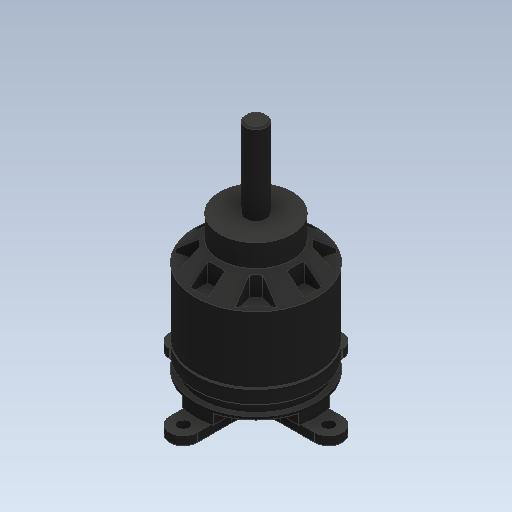
# Autodesk Inventor part: CobraCP2814-1050kv
Saved by Autodesk Inventor 2020 (Build 240168000, 168)
## iProperties
Part Number: CobraCP2814-1050kv
Material: GEDA Polyamid schwarz
Document SubType Name: Modeling
Designer: Admin
Mass: 32.8835 g
Surface Area: 99.7314 cm^2
Volume: 28.8452 cm^3
Density: 1.14 g/cm^3
Appearance: GEDA Plastik schwarz A
Gewicht: 0,033 kg
G_L: 0
G_H: 0
G_B: 0
InventorVersion: 2019.4
VAULT_Status: in Bearbeitung
Revision: -
Max. Breite: 0
Max. Höhe: 0
Max. Länge: 0
Max. Abmessungen: 0 x 0 x 0
Author: Admin
Autodesk Inventor part; units mm, degrees
note: some values were not read from the file. Left out: dimensions or parameters whose unit could not be read.
ref_plane "YZ Plane" through (0, 0, 0) normal (1, 0, 0) x (0, 1, 0)
ref_plane "XZ Plane" through (0, 0, 0) normal (0, 1, 0) x (-1, 0, 0)
ref_plane "XY Plane" through (0, 0, 0) normal (0, 0, 1) x (1, 0, 0)
sketch "Skizze1" plane through (0, 0, 0) normal (0, 0, 1) x (1, 0, 0)
  circle A0 centre (0, 0) radius 17.5
  dimension "d0" = 35
  constraints: 1 centre point, 1 coincident
  measures "d0" diameter of A0
extrude "Extrusion1" add sketch "Skizze1" along normal blind 36
sketch "Skizze3" plane through (0, 0, 36) normal (0, 0, 1) x (1, 0, 0)
  circle A0 centre (0, 0) radius 10.5
  dimension "d11" = 21
  constraints: 1 centre point, 1 coincident
  measures "d11" diameter of A0
chamfer "Fase2" distance 7 angle 40 1 edges at (-17.5, 0, 36) measured on face at (4.865, -5.1831, 36)
extrude "Extrusion2" add sketch "Skizze3" along normal blind 6.5
sketch "Skizze4" plane through (0, 0, 42.5) normal (0, 0, 1) x (1, 0, 0)
  circle A0 centre (0, 0) radius 3
  dimension "d17" = 6
  constraints: 1 centre point, 1 coincident
  measures "d17" diameter of A0
extrude "Extrusion3" add sketch "Skizze4" along normal blind 23.5
chamfer "Fase3" distance 0.5 angle 45 1 edges at (-3, 0, 66)
sketch "Skizze2" plane through (0, 0, 0) normal (1, 0, 0) x (0, 1, 0)
  line L0 (17.5, 11.1263) -> (16.5, 11.1263)
  line L1 (16.5, 11.1263) -> (16.5, 10.6263)
  line L2 (16.5, 10.6263) -> (17.5, 10.6263)
  line L3 (17.5, 10.6263) -> (17.5, 11.1263)
  line L4 (-17.5, 0) -> (17.5, 0) projected
  line L5 (17.5, 30.1263) -> (-17.5, 30.1263) projected
  point P0 (0, 0)
  point P1 (-17.5, 32)
  dimension "d6" = 1
  dimension "d7" = 0.5
  dimension "d23" = 19
  constraints: 8 end point, 2 parallel, 1 horizontal, 1 perpendicular, 1 point on line
  measures "d6" distance of L2.end L1.end
  measures "d7" distance of L1.end L0.end
  measures "d23" distance from line of L5 L0.start
sketch3d "3D-Skizze2"
  arc A0 (17.5, 0, 0) -> (0, -17.5, 0) centre (0, 0, 0) ccw
  arc A1 (0, -17.5, 0) -> (-17.5, 0, 0) centre (0, 0, 0) ccw
  arc A2 (-17.5, 0, 0) -> (0, 17.5, 0) centre (0, 0, 0) ccw
  arc A3 (0, 17.5, 0) -> (17.5, 0, 0) centre (0, 0, 0) ccw
sweep "Sweeping2" cut profiles "Skizze2" path "3D-Skizze2"
sketch "Skizze5" plane through (0, 0, 0) normal (0, 0, -1) x (-1, 0, 0)
  circle A0 centre (0, 0) radius 12.5 construction
  circle A1 centre (0, 12.5) radius 1.5
  circle A2 centre (12.5, 0) radius 1.5
  circle A3 centre (0, -12.5) radius 1.5
  circle A4 centre (-12.5, 0) radius 1.5
  dimension "d26" = 25
  dimension "d27" = 3
  constraints: 5 centre point, 4 point on circle, 3 equal radius, 2 horizontal alignment, 2 vertical alignment, 1 coincident
  measures "d26" diameter of A0
  measures "d27" diameter of A1
extrude "Extrusion4" cut sketch "Skizze5" against normal blind 5
sketch "Skizze6" plane through (0, 0, 0) normal (0, 0, -1) x (-1, 0, 0)
  line L0 (-4.5, -17.5) -> (4.5, -17.5) construction
  line L1 (4.5, -17.5) -> (4.5, 17.5) construction
  line L2 (4.5, 17.5) -> (-4.5, 17.5) construction
  line L3 (-4.5, 17.5) -> (-4.5, -17.5) construction
  line L4 (-4.5, -17.5) -> (4.5, 17.5) construction
  line L5 (4.5, -17.5) -> (-4.5, 17.5) construction
  line L6 (-17.5, -4.5) -> (17.5, -4.5) construction
  line L7 (17.5, -4.5) -> (17.5, 4.5) construction
  line L8 (17.5, 4.5) -> (-17.5, 4.5) construction
  line L9 (-17.5, 4.5) -> (-17.5, -4.5) construction
  line L10 (-17.5, -4.5) -> (17.5, 4.5) construction
  line L11 (17.5, -4.5) -> (-17.5, 4.5) construction
  circle A0 centre (0, 0) radius 17.5 projected
  circle A1 centre (0, 12.5) radius 1.5 construction
  circle A2 centre (12.5, 0) radius 1.5 construction
  circle A3 centre (0, -12.5) radius 1.5 construction
  circle A4 centre (-12.5, 0) radius 1.5 construction
  line L12 (0, -12.5) -> (12.5, 0) construction
  line L13 (12.5, 0) -> (0, 12.5) construction
  line L14 (0, 12.5) -> (-12.5, 0) construction
  line L15 (-12.5, 0) -> (0, -12.5) construction
  line L16 (0, -12.5) -> (0, 12.5) construction
  line L17 (12.5, 0) -> (-12.5, 0) construction
  circle A5 centre (0, 0) radius 17.5
  line L18 (-4.5, 16.9115) -> (-4.5, 8)
  line L19 (-4.5, 8) -> (-8, 4.5)
  line L20 (-16.9115, 4.5) -> (-8, 4.5)
  line L21 (4.5, 16.9115) -> (4.5, 8)
  line L22 (8, 4.5) -> (4.5, 8)
  line L23 (8, 4.5) -> (16.9115, 4.5)
  line L24 (-16.9115, -4.5) -> (-8, -4.5)
  line L25 (-8, -4.5) -> (-4.5, -8)
  line L26 (-4.5, -8) -> (-4.5, -16.9115)
  line L27 (4.5, -16.9115) -> (4.5, -8)
  line L28 (8, -4.5) -> (4.5, -8)
  line L29 (8, -4.5) -> (16.9115, -4.5)
  dimension "d31" = 9
  dimension "d32" = 9
  constraints: 60 end point, 24 point on line, 6 midpoint, 6 parallel, 4 perpendicular, 3 coincident, 2 collinear, 2 horizontal, 2 tangent, 11 other
  measures "d31" distance of L2.end L1.end
  measures "d32" distance of L7.end L6.end
extrude "Extrusion5" cut sketch "Skizze6" against normal blind 3 contours L23 L22 L21 A0 | A0 L27 L28 L29 | L18 L19 L20 A0 | A0 L24 L25 L26
fillet "Rundung1" radius 3 8 edges at (-8, 4.5, 1.5) (-4.5, 8, 1.5) (-8, -4.5, 1.5) (-4.5, -8, 1.5) (4.5, -8, 1.5) (8, -4.5, 1.5) (8, 4.5, 1.5) (4.5, 8, 1.5)
sketch "Skizze7" plane through (0, 0, 0) normal (1, 0, 0) x (0, 1, 0)
  line L0 (0, 1.5) -> (0, 10.6263)
  line L1 (0, 10.6263) -> (14.5, 10.6263)
  line L2 (9.2426, 3) -> (16.9115, 3) projected
  line L3 (14.5, 10.6263) -> (14.5, 1.5)
  line L4 (14.5, 1.5) -> (0, 1.5)
  line L5 (16.9115, 0) -> (9.2426, 0) projected
  line L6 (7.1213, 0) -> (9.2426, 0) projected
  line L7 (7.1213, 0) -> (5.3787, 0) projected
  line L8 (4.5, 0) -> (5.3787, 0) projected
  line L9 (-5.3787, 0) -> (-4.5, 0) projected
  line L10 (-5.3787, 0) -> (-7.1213, 0) projected
  line L11 (-9.2426, 0) -> (-7.1213, 0) projected
  line L12 (-9.2426, 0) -> (-16.9115, 0) projected
  line L13 (-16.9115, 0) -> (-9.2426, 0) projected
  line L14 (-7.1213, 0) -> (-9.2426, 0) projected
  line L15 (-7.1213, 0) -> (-5.3787, 0) projected
  line L16 (-4.5, 0) -> (-5.3787, 0) projected
  line L17 (5.3787, 0) -> (4.5, 0) projected
  line L18 (5.3787, 0) -> (7.1213, 0) projected
  line L19 (9.2426, 0) -> (7.1213, 0) projected
  line L20 (9.2426, 0) -> (16.9115, 0) projected
  line L21 (1.5, 0) -> (-1.5, 0) projected
  line L22 (1.5, 0) -> (-1.5, 0) projected
  line L23 (14, 0) -> (11, 0) projected
  line L24 (-11, 0) -> (-14, 0) projected
  line L25 (-17.5, 10.6263) -> (17.5, 10.6263) projected
  line L26 (-16.9115, 0) -> (-16.9115, 0) projected
  line L27 (-4.5, 0) -> (4.5, 0) projected
  line L28 (16.9115, 0) -> (16.9115, 0) projected
  line L29 (4.5, 0) -> (-4.5, 0) projected
  line L30 (17.5, 0) -> (17.5, 10.6263) projected
  line L31 (16, 3.8132) -> (17.5, 3.8132)
  line L32 (17.5, 3.8132) -> (17.5, 6.8132)
  line L33 (17.5, 6.8132) -> (16, 6.8132)
  line L34 (16, 6.8132) -> (16, 3.8132)
  line L35 (16, 3.8132) -> (17.5, 6.8132) construction
  line L36 (17.5, 3.8132) -> (16, 6.8132) construction
  point P0 (0, 0)
  point P1 (16.691, 9)
  point P2 (16.75, 5.3132)
  point P3 (16.75, 5.3132)
  point P4 (17.5, 5.3132)
  dimension "d41" = 1.5
  dimension "d75" = 3
  dimension "d76" = 1.5
  dimension "d77" = 3
  constraints: 20 end point, 4 midpoint, 4 parallel, 2 collinear, 2 horizontal, 1 horizontal alignment, 1 perpendicular, 1 point on line, 1 vertical, 1 other
  measures "d41" distance between parallel lines of L19 L4
  measures "d75" distance between parallel lines of L3 L30
  measures "d76" distance of L33.end L32.end
  measures "d77" distance of L33.end L31.start
revolve "Umdrehung1" cut sketch "Skizze7" angle 360 about axis through (0, 0, 1.5) along (0, 0, 1)
sketch "Skizze8" plane through (0, 0, 42.5) normal (0, 0, 1) x (1, 0, 0)
  circle A0 centre (0, 0) radius 17.5 projected
  circle A1 centre (0, 0) radius 10.5 projected
  line L0 (-2.5, 11.5) -> (2.5, 11.5)
  line L1 (2.5, 11.5) -> (2.5, 16.5)
  line L2 (2.5, 16.5) -> (-2.5, 16.5)
  line L3 (-2.5, 16.5) -> (-2.5, 11.5)
  line L4 (-2.5, 11.5) -> (2.5, 16.5) construction
  line L5 (2.5, 11.5) -> (-2.5, 16.5) construction
  line L6 (8.626, 14.7085) -> (14.7085, 8.626)
  line L7 (14.7085, 8.626) -> (9.1317, 7.1317)
  line L8 (9.1317, 7.1317) -> (7.1317, 9.1317)
  line L9 (7.1317, 9.1317) -> (8.626, 14.7085)
  line L10 (0, 0) -> (8.1317, 8.1317) construction
  line L11 (0, 0) -> (0, 14) construction
  dimension "d11" = 21
  dimension "d43" = 14
  dimension "d44" = 5
  dimension "d45" = 5
  dimension "d46" = 30
  dimension "d47" = 45
  dimension "d48" = 11.5
  dimension "d49" = 11.5
  dimension "d50" = 16.5
  dimension "d51" = 16.5
  dimension "d78" = 2
  constraints: 24 end point, 3 midpoint, 2 parallel, 2 perpendicular, 1 coincident, 1 horizontal, 1 vertical, 1 other
  measures "d43" distance of point (0, 0) L11.end
  measures "d44" distance of L0.end L1.end
  measures "d45" distance of L0.start L0.end
  measures "d46" angle of L9 L10
  measures "d47" angle of L11 L10
  measures "d48" distance from line of point (0, 0) L0
  measures "d49" distance from line of L8 point (0, 0)
  measures "d50" distance from line of L2 point (0, 0)
  measures "d51" distance from line of point (0, 0) L6
  measures "d78" horizontal distance of L7.end L8.end
extrude "Extrusion6" cut sketch "Skizze8" against normal blind 13 contours L3 L2 L1 L0 | L6 L7 L8 L9
pattern_circular "Runde Anordnung1" count 4 over 360 about axis through (0, 0, -10) along (0, 0, 1) of "Extrusion6"
sketch "Skizze9" plane through (0, 0, 0) normal (0, 0, -1) x (-1, 0, 0)
  line L0 (-4, 25) -> (4, 25)
  line L1 (4, 25) -> (4, -25)
  line L2 (4, -25) -> (-4, -25)
  line L3 (-4, -25) -> (-4, 25)
  line L4 (-4, 25) -> (4, -25) construction
  line L5 (4, 25) -> (-4, -25) construction
  line L6 (-25, 4) -> (25, 4)
  line L7 (25, 4) -> (25, -4)
  line L8 (25, -4) -> (-25, -4)
  line L9 (-25, -4) -> (-25, 4)
  line L10 (-25, 4) -> (25, -4) construction
  line L11 (25, 4) -> (-25, -4) construction
  circle A0 centre (21, 0) radius 1.65
  circle A1 centre (0, 21) radius 1.65
  circle A2 centre (-21, 0) radius 1.65
  circle A3 centre (0, -21) radius 1.65
  line L12 (21, 0) -> (0, -21) construction
  line L13 (0, 21) -> (-21, 0) construction
  circle A4 centre (0, 12.5) radius 1.5 projected
  circle A5 centre (12.5, 0) radius 1.5 projected
  circle A6 centre (0, -12.5) radius 1.5 projected
  circle A7 centre (-12.5, 0) radius 1.5 projected
  point P0 (0, 0)
  dimension "d57" = 8
  dimension "d58" = 50
  dimension "d59" = 50
  dimension "d60" = 8
  dimension "d61" = 3.3
  dimension "d64" = 360
  dimension "d67" = 42
  constraints: 28 end point, 4 centre point, 4 midpoint, 4 parallel, 2 horizontal, 2 perpendicular, 9 other
  measures "d57" distance of L1.end L2.end
  measures "d58" distance of L0.end L1.end
  measures "d59" distance of L7.end L8.end
  measures "d60" distance of L6.end L7.end
  measures "d61" diameter of A0
  measures "d67" distance of L13.end L12.start
extrude "Extrusion7" add sketch "Skizze9" along normal blind 2.5
fillet "Rundung3" radius 7 4 edges at (-4, -4, -1.25) (-4, 4, -1.25) (4, 4, -1.25) (4, -4, -1.25)
fillet "Rundung4" radius 4 8 edges at (-25, -4, -1.25) (-25, 4, -1.25) (-4, -25, -1.25) (4, -25, -1.25) (25, -4, -1.25) (25, 4, -1.25) (4, 25, -1.25) (-4, 25, -1.25)
sketch "Skizze10" plane through (0, 0, -2.5) normal (0, 0, -1) x (-1, 0, 0)
  circle A0 centre (0, 0) radius 6
  dimension "d72" = 12
  constraints: 1 centre point, 1 coincident
  measures "d72" diameter of A0
extrude "Extrusion8" cut sketch "Skizze10" against normal blind 2.5
equation "\"d41\" = d40"
equation "\"d49\" = d48"
equation "\"d51\" = d50"
equation "\"G_L\" = 0"
equation "\"G_H\" = 0"
equation "\"G_B\" = 0"
equation "\"d40\" = 1.5"
